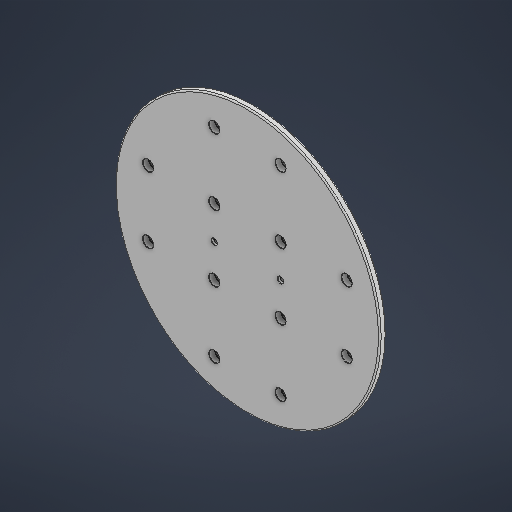
# Autodesk Inventor part: tableStandBottom
Saved by Autodesk Inventor 2026.3 (Build 303398000, 398)
## iProperties
Created: 2026-06-26
Part Number: tableStandBottom
Material: Generic
Document SubType Name: Modeling
Designer: frede
Density: 1 g/cm^3
Appearance: Default
Author: frede
Autodesk Inventor part; units mm, degrees
ref_plane "YZ Plane" through (0, 0, 0) normal (1, 0, 0) x (0, 1, 0)
ref_plane "XZ Plane" through (0, 0, 0) normal (0, 1, 0) x (-1, 0, 0)
ref_plane "XY Plane" through (0, 0, 0) normal (0, 0, 1) x (1, 0, 0)
sketch "Sketch1" plane through (0, 0, 0) normal (0, 0, 1) x (1, 0, 0)
  circle A0 centre (0, 0) radius 100
  line L0 (25, 25) -> (-25, 25)
  line L1 (-25, 25) -> (-25, -25)
  line L2 (-25, -25) -> (25, -25)
  line L3 (25, -25) -> (25, 25)
  line L4 (25, 25) -> (-25, -25) construction
  line L5 (-25, 25) -> (25, -25) construction
  line L6 (25, 25) -> (-25, 25)
  line L7 (-25, 25) -> (-25, 75)
  line L8 (-25, 75) -> (25, 75)
  line L9 (25, 75) -> (25, 25)
  line L10 (-25, 25) -> (-75, 25)
  line L11 (-75, 25) -> (-75, -25)
  line L12 (-75, -25) -> (-25, -25)
  line L13 (-25, -25) -> (-25, 25)
  line L14 (-25, 25) -> (-75, 25)
  line L15 (-75, 25) -> (-75, 75)
  line L16 (-75, 75) -> (-25, 75)
  line L17 (-25, 75) -> (-25, 25)
  line L18 (-75, -25) -> (-25, -25)
  line L19 (-25, -25) -> (-25, -75)
  line L20 (-25, -75) -> (-75, -75)
  line L21 (-75, -75) -> (-75, -25)
  line L22 (-25, -75) -> (25, -75)
  line L23 (25, -75) -> (25, -25)
  line L24 (25, -25) -> (-25, -25)
  line L25 (-25, -25) -> (-25, -75)
  line L26 (25, -25) -> (75, -25)
  line L27 (75, -25) -> (75, -75)
  line L28 (75, -75) -> (25, -75)
  line L29 (25, -75) -> (25, -25)
  line L30 (75, -25) -> (25, -25)
  line L31 (25, -25) -> (25, 25)
  line L32 (25, 25) -> (75, 25)
  line L33 (75, 25) -> (75, -25)
  line L34 (25, 25) -> (75, 25)
  line L35 (75, 25) -> (75, 75)
  line L36 (75, 75) -> (25, 75)
  line L37 (25, 75) -> (25, 25)
  circle A1 centre (75, 25) radius 7.9
  circle A2 centre (25, 75) radius 7.9
  circle A3 centre (-25, 75) radius 7.9
  circle A4 centre (25, 25) radius 7.9
  circle A5 centre (-25, 25) radius 7.9
  circle A6 centre (-75, 25) radius 7.9
  circle A7 centre (-75, -25) radius 7.9
  circle A8 centre (-25, -25) radius 7.9
  circle A9 centre (25, -25) radius 7.9
  circle A10 centre (75, -25) radius 7.9
  circle A11 centre (25, -75) radius 7.9
  circle A12 centre (-25, -75) radius 7.9
  dimension "d0" = 200
  dimension "d12" = 50
  dimension "d14" = 50
  dimension "d15" = 15.8
  dimension "d16" = 15.8
  dimension "d17" = 15.8
  dimension "d18" = 15.8
  dimension "d19" = 15.8
  dimension "d20" = 15.8
  dimension "d22" = 15.8
  dimension "d23" = 15.8
  dimension "d24" = 15.8
  dimension "d25" = 15.8
  dimension "d26" = 15.8
  dimension "d27" = 15.8
  dimension "d30" = 50
  dimension "d31" = 50
  dimension "d32" = 50
  dimension "d33" = 50
  constraints: 76 end point, 18 parallel, 13 centre point, 13 coincident, 9 horizontal, 9 perpendicular, 2 midpoint, 2 point on line
  measures "d0" diameter of A0
  measures "d12" distance of L19.end L20.end
  measures "d14" distance of L27.end L28.end
  measures "d15" diameter of A1
  measures "d16" diameter of A2
  measures "d17" diameter of A3
  measures "d18" diameter of A4
  measures "d19" diameter of A5
  measures "d20" diameter of A6
  measures "d22" diameter of A7
  measures "d23" diameter of A8
  measures "d24" diameter of A9
  measures "d25" diameter of A10
  measures "d26" diameter of A11
  measures "d27" diameter of A12
  measures "d30" distance between parallel lines of L19 L23
  measures "d31" distance between parallel lines of L26 L28
  measures "d32" distance between parallel lines of L26 L32
  measures "d33" distance between parallel lines of L32 L36
extrude "Extrusion1" add sketch "Sketch1" along normal blind 5 contours A0 L27 A10 L33 A1 L35 | L35 A1 L32 A4 L9 A2 L36 A0 | A0 L28 A11 L23 A9 L26 A10 L27 | L36 A2 L8 A3 L16 A0 | A1 L33 L35 | L35 L32 A1 | A0 L20 A12 L22 A11 L28 | A10 L26 L27 | L27 L33 A10 | L16 A3 L7 A5 L10 A6 L15 A0 | A2 L9 L36 | L36 L8 A2 | L33 A1 L32 | A1 L33 A10 L26 A9 L3 A4 L32 | A0 L21 A7 L12 A8 L19 A12 L20 | A11 L22 L28 | L28 L23 A11 | L26 A10 L33 | L15 A6 L11 A7 L21 A0 | A3 L8 L16 | L16 L7 A3 | L9 A2 L8 | A2 L9 A4 L0 A5 L7 A3 L8 | A4 L3 L32 | L32 L9 A4 | A12 L19 L20 | L20 L22 A12 | L22 A11 L23 | A11 L22 A12 L19 A8 L2 A9 L23 | A9 L23 L26 | L26 L3 A9 | A6 L10 L15 | L15 L11 A6 | L8 A3 L7 | L9 L0 A4 | L3 A4 L0 | L3 A9 L2 A8 L1 A5 L0 A4 | A7 L11 L21 | L21 L12 A7 | L19 A12 L22 | A9 L2 L23 | L2 A9 L3 | L10 A6 L11 | L10 A5 L1 A8 L12 A7 L11 A6 | A5 L0 L7 | L7 L10 A5 | L11 A7 L12 | A8 L12 L19 | L19 L2 A8 | L10 L1 A5 | L0 A5 L1 | A8 L1 L12 | L1 A8 L2
extrude "Extrusion2" add sketch "Sketch1" against normal blind 8 contours A1 L33 L35 | L35 L32 A1 | A10 L26 L27 | L27 L33 A10 | A2 L9 L36 | L36 L8 A2 | L33 A1 L32 | A11 L22 L28 | L28 L23 A11 | L26 A10 L33 | A3 L8 L16 | L16 L7 A3 | L9 A2 L8 | A4 L3 L32 | L32 L9 A4 | A12 L19 L20 | L20 L22 A12 | L22 A11 L23 | A9 L23 L26 | L26 L3 A9 | A6 L10 L15 | L15 L11 A6 | L8 A3 L7 | L9 L0 A4 | L3 A4 L0 | A7 L11 L21 | L21 L12 A7 | L19 A12 L22 | A9 L2 L23 | L2 A9 L3 | L10 A6 L11 | A5 L0 L7 | L7 L10 A5 | L11 A7 L12 | A8 L12 L19 | L19 L2 A8 | L10 L1 A5 | L0 A5 L1 | A8 L1 L12 | L1 A8 L2
fillet "Fillet1" radius 1 26 edges at (17.1, 75, 0) (-32.9, 75, 0) (-82.9, 25, 0) (-32.9, 25, 0) (17.1, 25, 0) (67.1, 25, 0) (67.1, -25, 0) (17.1, -25, 0) (-32.9, -25, 0) (-82.9, -25, 0) (-32.9, -75, 0) (17.1, -75, 0) (17.1, -75, -8) (-32.9, -75, -8) (-32.9, -25, -8) (-82.9, -25, -8) (17.1, -25, -8) (67.1, -25, -8) (67.1, 25, -8) (17.1, 25, -8) (-32.9, 25, -8) (-82.9, 25, -8) (-32.9, 75, -8) (17.1, 75, -8) (-100, 0, 0) (-100, 0, 5)
sketch "Sketch2" plane through (0, 0, 0) normal (0, 0, -1) x (-1, 0, 0)
  circle A0 centre (-25, 0) radius 2.2
  circle A1 centre (25, 0) radius 2.2
  point P0 (0, 0)
  dimension "d37" = 4.4
  dimension "d38" = 4.4
  dimension "d39" = 50
  dimension "d40" = 25
  constraints: 2 centre point
  measures "d37" diameter of A0
  measures "d38" diameter of A1
  measures "d39" distance of A1.centre A0.centre
  measures "d40" distance of point (0, 0) A0.centre
extrude "Extrusion3" cut sketch "Sketch2" against normal up to surface (5 mm away)
sketch "Sketch3" plane through (0, 0, 0) normal (0, 0, -1) x (-1, 0, 0)
  circle A0 centre (-25, 0) radius 2.2 projected
  line L0 (-21.4, -2.0785) -> (-25, -4.1569)
  line L1 (-25, -4.1569) -> (-28.6, -2.0785)
  line L2 (-28.6, -2.0785) -> (-28.6, 2.0785)
  line L3 (-28.6, 2.0785) -> (-25, 4.1569)
  line L4 (-25, 4.1569) -> (-21.4, 2.0785)
  line L5 (-21.4, 2.0785) -> (-21.4, -2.0785)
  circle A1 centre (25, 0) radius 2.2 projected
  line L6 (28.6, -2.0785) -> (25, -4.1569)
  line L7 (25, -4.1569) -> (21.4, -2.0785)
  line L8 (21.4, -2.0785) -> (21.4, 2.0785)
  line L9 (21.4, 2.0785) -> (25, 4.1569)
  line L10 (25, 4.1569) -> (28.6, 2.0785)
  line L11 (28.6, 2.0785) -> (28.6, -2.0785)
  point P0 (0, 0)
  dimension "d43" = 7.2
  dimension "d44" = 7.2
  constraints: 24 end point, 2 coincident, 26 other
  measures "d43" distance between parallel lines of L5 L2
  measures "d44" distance between parallel lines of L11 L8
extrude "Extrusion4" cut sketch "Sketch3" against normal blind 3 contours A0 | L0 L1 L2 L3 L4 L5 | A1 | L6 L7 L8 L9 L10 L11
sketch "Sketch4" plane through (25, -25, -8) normal (0, 0, -1) x (-1, 0, 0)
  circle A0 centre (0, 0) radius 8.9 projected
  circle A1 centre (0, 50) radius 7.9 projected
  circle A2 centre (50, 50) radius 7.9 projected
  circle A3 centre (50, 0) radius 6.9 projected
  circle A4 centre (-50, 0) radius 7.9 projected
  circle A5 centre (-50, 50) radius 7.9 projected
  circle A6 centre (0, 100) radius 7.9 projected
  circle A7 centre (50, 100) radius 6.9 projected
  circle A8 centre (100, 50) radius 6.9 projected
  circle A9 centre (100, 0) radius 6.9 projected
  circle A10 centre (50, -50) radius 6.9 projected
  circle A11 centre (0, -50) radius 6.9 projected
  point P0 (25, 25)
  constraints: 12 coincident
hole "Hole1" at (25, -25, -8) at (25, 25, -8) at (-25, 25, -8) at (-25, -25, -8) at (25, -75, -8) at (-25, -75, -8) at (-75, -25, -8) at (-75, 25, -8) at (-25, 75, -8) at (25, 75, -8) at (75, 25, -8) at (75, -25, -8) direction (0, 0, 1) diameter 4.4 depth 13 tip angle 118 countersink diameter 6 countersink angle 90
sketch "Sketch5" plane through (0, 0, 5) normal (0, 0, 1) x (1, 0, 0)
  circle A0 centre (25, 25) radius 2.2 projected
  circle A1 centre (25, 25) radius 4
  circle A2 centre (25, -25) radius 2.2 projected
  circle A3 centre (25, -25) radius 4
  circle A4 centre (-25, -25) radius 2.2 projected
  circle A5 centre (-25, -25) radius 4
  circle A6 centre (-25, 25) radius 2.2 projected
  circle A7 centre (-25, 25) radius 4
  circle A8 centre (25, -75) radius 2.2 projected
  circle A9 centre (25, -75) radius 4
  circle A10 centre (-25, -75) radius 2.2 projected
  circle A11 centre (-25, -75) radius 4
  circle A12 centre (75, -25) radius 4
  circle A13 centre (75, 25) radius 4
  circle A14 centre (25, 75) radius 4
  circle A15 centre (-25, 75) radius 4
  circle A16 centre (-75, 25) radius 4
  circle A17 centre (-75, -25) radius 4
  point P0 (0, 0)
  dimension "d55" = 8
  dimension "d56" = 8
  dimension "d57" = 8
  dimension "d58" = 8
  dimension "d62" = 8
  dimension "d63" = 8
  dimension "d66" = 360
  constraints: 12 centre point, 6 coincident, 17 other
  measures "d55" diameter of A1
  measures "d56" diameter of A3
  measures "d57" diameter of A5
  measures "d58" diameter of A7
  measures "d62" diameter of A9
  measures "d63" diameter of A11
extrude "Extrusion5" cut sketch "Sketch5" against normal blind 4.5 contours A0 | A1 | A2 | A3 | A4 | A5 | A6 | A7 | A8 | A9 | A10 | A11 | A12 | A13 | A14 | A15 | A16 | A17
fillet "Fillet2" radius 0.25 76 edges at (27.2, 0, 3) (27.2, 0, 5) (23.2, 3.1177, 3) (21.4, 0, 3) (23.2, -3.1177, 3) (26.8, -3.1177, 3) (28.6, 0, 3) (26.8, 3.1177, 3) (26.8, 3.1177, 0) (23.2, 3.1177, 0) (21.4, 0, 0) (23.2, -3.1177, 0) (26.8, -3.1177, 0) (28.6, 0, 0) (-28.6, 0, 0) (-26.8, 3.1177, 0) (-23.2, 3.1177, 0) (-21.4, 0, 0) (-23.2, -3.1177, 0) (-26.8, -3.1177, 0) (-28.6, 0, 3) (-26.8, 3.1177, 3) (-23.2, 3.1177, 3) (-21.4, 0, 3) (-23.2, -3.1177, 3) (-26.8, -3.1177, 3) (-22.8, 0, 3) (-22.8, 0, 5) (21, 25, 5) (25, 22.8, 0.5) (-29, 25, 5) (-25, 22.8, 0.5) (-25, 22.8, -7.2) (25, 22.8, -7.2) (25, -27.2, -7.2) (25, -27.2, 0.5) (21, -25, 5) (-29, -25, 5) (-25, -27.2, 0.5) (-25, -27.2, -7.2) (-29, -25, 0.5) (21, -25, 0.5) (21, 25, 0.5) (-29, 25, 0.5) (-29, -75, 5) (-25, -77.2, 0.5) (-29, -75, 0.5) (-25, -77.2, -7.2) (21, -75, 5) (21, -75, 0.5) (25, -77.2, 0.5) (25, -77.2, -7.2) (71, -25, 5) (71, -25, 0.5) (75, -27.2, 0.5) (75, -27.2, -7.2) (71, 25, 5) (71, 25, 0.5) (75, 22.8, 0.5) (75, 22.8, -7.2) (21, 75, 5) (21, 75, 0.5) (25, 72.8, 0.5) (25, 72.8, -7.2) (-29, 75, 5) (-29, 75, 0.5) (-25, 72.8, 0.5) (-25, 72.8, -7.2) (-79, 25, 5) (-79, 25, 0.5) (-75, 22.8, 0.5) (-75, 22.8, -7.2) (-79, -25, 5) (-79, -25, 0.5) (-75, -27.2, 0.5) (-75, -27.2, -7.2)
equation "\"d16\" = d15"
equation "\"d17\" = d15"
equation "\"d18\" = d15"
equation "\"d19\" = d15"
equation "\"d20\" = d15"
equation "\"d22\" = d15"
equation "\"d23\" = d15"
equation "\"d24\" = d15"
equation "\"d25\" = d15"
equation "\"d26\" = d15"
equation "\"d27\" = d15"
equation "\"d38\" = d37"
equation "\"d56\" = d55"
equation "\"d57\" = d55"
equation "\"d58\" = d55"
equation "\"d62\" = d63"
body "Solid1"
